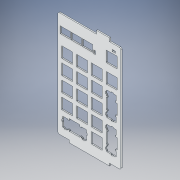
# Autodesk Inventor part: NumpadPlate
Saved by Autodesk Inventor 2018 (Build 220112000, 112)
## iProperties
Created: 2024-10-28
Part Number: NumpadPlate
Material: Generic
Document SubType Name: Modeling
Designer: yuchi
Density: 1 g/cm^3
Appearance: White
Author: yuchi
Autodesk Inventor part; units mm, degrees
ref_plane "YZ Plane" through (0, 0, 0) normal (1, 0, 0) x (0, 1, 0)
ref_plane "XZ Plane" through (0, 0, 0) normal (0, 1, 0) x (-1, 0, 0)
ref_plane "XY Plane" through (0, 0, 0) normal (0, 0, 1) x (1, 0, 0)
sketch "0" plane through (0, 0, 0) normal (0, 0, 1) x (1, 0, 0)
  line L0 (0.6438, 2.2375) -> (13.6438, 2.2375)
  line L1 (0.6438, -11.7625) -> (13.6438, -11.7625)
  line L2 (0.1438, 1.7375) -> (0.1438, -11.2625)
  line L3 (14.1438, 1.7375) -> (14.1438, -11.2625)
  arc A0 (0.6438, 2.2375) -> (0.1438, 1.7375) centre (0.6438, 1.7375) ccw
  arc A1 (14.1438, 1.7375) -> (13.6438, 2.2375) centre (13.6438, 1.7375) ccw
  arc A2 (0.1438, -11.2625) -> (0.6438, -11.7625) centre (0.6438, -11.2625) ccw
  arc A3 (13.6438, -11.7625) -> (14.1438, -11.2625) centre (13.6438, -11.2625) ccw
  line L4 (14.9313, 2.2375) -> (27.9312, 2.2375)
  line L5 (14.9313, -11.7625) -> (27.9312, -11.7625)
  line L6 (14.4313, 1.7375) -> (14.4313, -11.2625)
  line L7 (28.4313, 1.7375) -> (28.4313, -11.2625)
  arc A4 (14.9313, 2.2375) -> (14.4313, 1.7375) centre (14.9313, 1.7375) ccw
  arc A5 (28.4313, 1.7375) -> (27.9312, 2.2375) centre (27.9312, 1.7375) ccw
  arc A6 (14.4313, -11.2625) -> (14.9313, -11.7625) centre (14.9313, -11.2625) ccw
  arc A7 (27.9312, -11.7625) -> (28.4313, -11.2625) centre (27.9312, -11.2625) ccw
  line L8 (29.2188, 2.2375) -> (42.2188, 2.2375)
  line L9 (29.2188, -11.7625) -> (42.2188, -11.7625)
  line L10 (28.7188, 1.7375) -> (28.7188, -11.2625)
  line L11 (42.7188, 1.7375) -> (42.7188, -11.2625)
  arc A8 (29.2188, 2.2375) -> (28.7188, 1.7375) centre (29.2188, 1.7375) ccw
  arc A9 (42.7188, 1.7375) -> (42.2188, 2.2375) centre (42.2188, 1.7375) ccw
  arc A10 (28.7188, -11.2625) -> (29.2188, -11.7625) centre (29.2188, -11.2625) ccw
  arc A11 (42.2188, -11.7625) -> (42.7188, -11.2625) centre (42.2188, -11.2625) ccw
  line L12 (3.025, -21.575) -> (16.025, -21.575)
  line L13 (3.025, -35.575) -> (16.025, -35.575)
  line L14 (2.525, -22.075) -> (2.525, -35.075)
  line L15 (16.525, -22.075) -> (16.525, -35.075)
  arc A12 (3.025, -21.575) -> (2.525, -22.075) centre (3.025, -22.075) ccw
  arc A13 (16.525, -22.075) -> (16.025, -21.575) centre (16.025, -22.075) ccw
  arc A14 (2.525, -35.075) -> (3.025, -35.575) centre (3.025, -35.075) ccw
  arc A15 (16.025, -35.575) -> (16.525, -35.075) centre (16.025, -35.075) ccw
  line L16 (22.075, -21.575) -> (35.075, -21.575)
  line L17 (22.075, -35.575) -> (35.075, -35.575)
  line L18 (21.575, -22.075) -> (21.575, -35.075)
  line L19 (35.575, -22.075) -> (35.575, -35.075)
  arc A16 (22.075, -21.575) -> (21.575, -22.075) centre (22.075, -22.075) ccw
  arc A17 (35.575, -22.075) -> (35.075, -21.575) centre (35.075, -22.075) ccw
  arc A18 (21.575, -35.075) -> (22.075, -35.575) centre (22.075, -35.075) ccw
  arc A19 (35.075, -35.575) -> (35.575, -35.075) centre (35.075, -35.075) ccw
  line L20 (41.125, -21.575) -> (54.125, -21.575)
  line L21 (41.125, -35.575) -> (54.125, -35.575)
  line L22 (40.625, -22.075) -> (40.625, -35.075)
  line L23 (54.625, -22.075) -> (54.625, -35.075)
  arc A20 (41.125, -21.575) -> (40.625, -22.075) centre (41.125, -22.075) ccw
  arc A21 (54.625, -22.075) -> (54.125, -21.575) centre (54.125, -22.075) ccw
  arc A22 (40.625, -35.075) -> (41.125, -35.575) centre (41.125, -35.075) ccw
  arc A23 (54.125, -35.575) -> (54.625, -35.075) centre (54.125, -35.075) ccw
  line L24 (60.175, -21.575) -> (73.175, -21.575)
  line L25 (60.175, -35.575) -> (73.175, -35.575)
  line L26 (59.675, -22.075) -> (59.675, -35.075)
  line L27 (73.675, -22.075) -> (73.675, -35.075)
  arc A24 (60.175, -21.575) -> (59.675, -22.075) centre (60.175, -22.075) ccw
  arc A25 (73.675, -22.075) -> (73.175, -21.575) centre (73.175, -22.075) ccw
  arc A26 (59.675, -35.075) -> (60.175, -35.575) centre (60.175, -35.075) ccw
  arc A27 (73.175, -35.575) -> (73.675, -35.075) centre (73.175, -35.075) ccw
  line L28 (3.025, -40.625) -> (16.025, -40.625)
  line L29 (3.025, -54.625) -> (16.025, -54.625)
  line L30 (2.525, -41.125) -> (2.525, -54.125)
  line L31 (16.525, -41.125) -> (16.525, -54.125)
  arc A28 (3.025, -40.625) -> (2.525, -41.125) centre (3.025, -41.125) ccw
  arc A29 (16.525, -41.125) -> (16.025, -40.625) centre (16.025, -41.125) ccw
  arc A30 (2.525, -54.125) -> (3.025, -54.625) centre (3.025, -54.125) ccw
  arc A31 (16.025, -54.625) -> (16.525, -54.125) centre (16.025, -54.125) ccw
  line L32 (22.075, -40.625) -> (35.075, -40.625)
  line L33 (22.075, -54.625) -> (35.075, -54.625)
  line L34 (21.575, -41.125) -> (21.575, -54.125)
  line L35 (35.575, -41.125) -> (35.575, -54.125)
  arc A32 (22.075, -40.625) -> (21.575, -41.125) centre (22.075, -41.125) ccw
  arc A33 (35.575, -41.125) -> (35.075, -40.625) centre (35.075, -41.125) ccw
  arc A34 (21.575, -54.125) -> (22.075, -54.625) centre (22.075, -54.125) ccw
  arc A35 (35.075, -54.625) -> (35.575, -54.125) centre (35.075, -54.125) ccw
  line L36 (41.125, -40.625) -> (54.125, -40.625)
  line L37 (41.125, -54.625) -> (54.125, -54.625)
  line L38 (40.625, -41.125) -> (40.625, -54.125)
  line L39 (54.625, -41.125) -> (54.625, -54.125)
  arc A36 (41.125, -40.625) -> (40.625, -41.125) centre (41.125, -41.125) ccw
  arc A37 (54.625, -41.125) -> (54.125, -40.625) centre (54.125, -41.125) ccw
  arc A38 (40.625, -54.125) -> (41.125, -54.625) centre (41.125, -54.125) ccw
  arc A39 (54.125, -54.625) -> (54.625, -54.125) centre (54.125, -54.125) ccw
  line L40 (73.675, -50.65) -> (73.675, -63.65)
  line L41 (59.675, -50.65) -> (59.675, -63.65)
  line L42 (73.175, -50.15) -> (60.175, -50.15)
  line L43 (73.175, -64.15) -> (60.175, -64.15)
  arc A40 (73.675, -50.65) -> (73.175, -50.15) centre (73.175, -50.65) ccw
  arc A41 (73.175, -64.15) -> (73.675, -63.65) centre (73.175, -63.65) ccw
  arc A42 (60.175, -50.15) -> (59.675, -50.65) centre (60.175, -50.65) ccw
  arc A43 (59.675, -63.65) -> (60.175, -64.15) centre (60.175, -63.65) ccw
  line L44 (72.3646, -42.3846) -> (72.3646, -48.0394)
  line L45 (71.8646, -48.5394) -> (71.5518, -48.5394)
  line L46 (71.5518, -48.5394) -> (71.5518, -57.15)
  line L47 (60.8584, -57.15) -> (60.8584, -49.0394)
  line L48 (60.3584, -48.5394) -> (60.071, -48.5394)
  line L49 (60.071, -48.5394) -> (60.071, -47.236)
  line L50 (59.571, -46.736) -> (59.4026, -46.736)
  line L51 (58.9026, -46.236) -> (58.9026, -44.188)
  line L52 (59.4026, -43.688) -> (59.571, -43.688)
  line L53 (60.071, -43.188) -> (60.071, -42.3846)
  line L54 (60.571, -41.8846) -> (65.667, -41.8846)
  line L55 (66.167, -41.3846) -> (66.167, -41.021)
  line L56 (66.167, -41.021) -> (68.461, -41.021)
  line L57 (68.961, -41.521) -> (68.961, -41.8846)
  line L58 (68.961, -41.8846) -> (71.8646, -41.8846)
  arc A44 (71.8646, -48.5394) -> (72.3646, -48.0394) centre (71.8646, -48.0394) ccw
  arc A45 (60.8584, -49.0394) -> (60.3584, -48.5394) centre (60.3584, -49.0394) ccw
  arc A46 (60.071, -47.236) -> (59.571, -46.736) centre (59.571, -47.236) ccw
  arc A47 (58.9026, -46.236) -> (59.4026, -46.736) centre (59.4026, -46.236) ccw
  arc A48 (59.4026, -43.688) -> (58.9026, -44.188) centre (59.4026, -44.188) ccw
  arc A49 (59.571, -43.688) -> (60.071, -43.188) centre (59.571, -43.188) ccw
  arc A50 (60.571, -41.8846) -> (60.071, -42.3846) centre (60.571, -42.3846) ccw
  arc A51 (65.667, -41.8846) -> (66.167, -41.3846) centre (65.667, -41.3846) ccw
  arc A52 (68.961, -41.521) -> (68.461, -41.021) centre (68.461, -41.521) ccw
  arc A53 (72.3646, -42.3846) -> (71.8646, -41.8846) centre (71.8646, -42.3846) ccw
  line L59 (72.3646, -71.9154) -> (72.3646, -66.2606)
  line L60 (71.8646, -65.7606) -> (71.5518, -65.7606)
  line L61 (71.5518, -65.7606) -> (71.5518, -57.15)
  line L62 (60.8584, -57.15) -> (60.8584, -65.2606)
  line L63 (60.3584, -65.7606) -> (60.071, -65.7606)
  line L64 (60.071, -65.7606) -> (60.071, -67.064)
  line L65 (59.571, -67.564) -> (59.4026, -67.564)
  line L66 (58.9026, -68.064) -> (58.9026, -70.112)
  line L67 (59.4026, -70.612) -> (59.571, -70.612)
  line L68 (60.071, -71.112) -> (60.071, -71.9154)
  line L69 (60.571, -72.4154) -> (65.667, -72.4154)
  line L70 (66.167, -72.9154) -> (66.167, -73.279)
  line L71 (66.167, -73.279) -> (68.461, -73.279)
  line L72 (68.961, -72.779) -> (68.961, -72.4154)
  line L73 (68.961, -72.4154) -> (71.8646, -72.4154)
  arc A54 (72.3646, -66.2606) -> (71.8646, -65.7606) centre (71.8646, -66.2606) ccw
  arc A55 (60.3584, -65.7606) -> (60.8584, -65.2606) centre (60.3584, -65.2606) ccw
  arc A56 (59.571, -67.564) -> (60.071, -67.064) centre (59.571, -67.064) ccw
  arc A57 (59.4026, -67.564) -> (58.9026, -68.064) centre (59.4026, -68.064) ccw
  arc A58 (58.9026, -70.112) -> (59.4026, -70.612) centre (59.4026, -70.112) ccw
  arc A59 (60.071, -71.112) -> (59.571, -70.612) centre (59.571, -71.112) ccw
  arc A60 (60.071, -71.9154) -> (60.571, -72.4154) centre (60.571, -71.9154) ccw
  arc A61 (66.167, -72.9154) -> (65.667, -72.4154) centre (65.667, -72.9154) ccw
  arc A62 (68.461, -73.279) -> (68.961, -72.779) centre (68.461, -72.779) ccw
  arc A63 (71.8646, -72.4154) -> (72.3646, -71.9154) centre (71.8646, -71.9154) ccw
  line L74 (3.025, -59.675) -> (16.025, -59.675)
  line L75 (3.025, -73.675) -> (16.025, -73.675)
  line L76 (2.525, -60.175) -> (2.525, -73.175)
  line L77 (16.525, -60.175) -> (16.525, -73.175)
  arc A64 (3.025, -59.675) -> (2.525, -60.175) centre (3.025, -60.175) ccw
  arc A65 (16.525, -60.175) -> (16.025, -59.675) centre (16.025, -60.175) ccw
  arc A66 (2.525, -73.175) -> (3.025, -73.675) centre (3.025, -73.175) ccw
  arc A67 (16.025, -73.675) -> (16.525, -73.175) centre (16.025, -73.175) ccw
  line L78 (22.075, -59.675) -> (35.075, -59.675)
  line L79 (22.075, -73.675) -> (35.075, -73.675)
  line L80 (21.575, -60.175) -> (21.575, -73.175)
  line L81 (35.575, -60.175) -> (35.575, -73.175)
  arc A68 (22.075, -59.675) -> (21.575, -60.175) centre (22.075, -60.175) ccw
  arc A69 (35.575, -60.175) -> (35.075, -59.675) centre (35.075, -60.175) ccw
  arc A70 (21.575, -73.175) -> (22.075, -73.675) centre (22.075, -73.175) ccw
  arc A71 (35.075, -73.675) -> (35.575, -73.175) centre (35.075, -73.175) ccw
  line L82 (41.125, -59.675) -> (54.125, -59.675)
  line L83 (41.125, -73.675) -> (54.125, -73.675)
  line L84 (40.625, -60.175) -> (40.625, -73.175)
  line L85 (54.625, -60.175) -> (54.625, -73.175)
  arc A72 (41.125, -59.675) -> (40.625, -60.175) centre (41.125, -60.175) ccw
  arc A73 (54.625, -60.175) -> (54.125, -59.675) centre (54.125, -60.175) ccw
  arc A74 (40.625, -73.175) -> (41.125, -73.675) centre (41.125, -73.175) ccw
  arc A75 (54.125, -73.675) -> (54.625, -73.175) centre (54.125, -73.175) ccw
  line L86 (3.025, -78.725) -> (16.025, -78.725)
  line L87 (3.025, -92.725) -> (16.025, -92.725)
  line L88 (2.525, -79.225) -> (2.525, -92.225)
  line L89 (16.525, -79.225) -> (16.525, -92.225)
  arc A76 (3.025, -78.725) -> (2.525, -79.225) centre (3.025, -79.225) ccw
  arc A77 (16.525, -79.225) -> (16.025, -78.725) centre (16.025, -79.225) ccw
  arc A78 (2.525, -92.225) -> (3.025, -92.725) centre (3.025, -92.225) ccw
  arc A79 (16.025, -92.725) -> (16.525, -92.225) centre (16.025, -92.225) ccw
  line L90 (22.075, -78.725) -> (35.075, -78.725)
  line L91 (22.075, -92.725) -> (35.075, -92.725)
  line L92 (21.575, -79.225) -> (21.575, -92.225)
  line L93 (35.575, -79.225) -> (35.575, -92.225)
  arc A80 (22.075, -78.725) -> (21.575, -79.225) centre (22.075, -79.225) ccw
  arc A81 (35.575, -79.225) -> (35.075, -78.725) centre (35.075, -79.225) ccw
  arc A82 (21.575, -92.225) -> (22.075, -92.725) centre (22.075, -92.225) ccw
  arc A83 (35.075, -92.725) -> (35.575, -92.225) centre (35.075, -92.225) ccw
  line L94 (41.125, -78.725) -> (54.125, -78.725)
  line L95 (41.125, -92.725) -> (54.125, -92.725)
  line L96 (40.625, -79.225) -> (40.625, -92.225)
  line L97 (54.625, -79.225) -> (54.625, -92.225)
  arc A84 (41.125, -78.725) -> (40.625, -79.225) centre (41.125, -79.225) ccw
  arc A85 (54.625, -79.225) -> (54.125, -78.725) centre (54.125, -79.225) ccw
  arc A86 (40.625, -92.225) -> (41.125, -92.725) centre (41.125, -92.225) ccw
  arc A87 (54.125, -92.725) -> (54.625, -92.225) centre (54.125, -92.225) ccw
  line L98 (73.675, -88.75) -> (73.675, -101.75)
  line L99 (59.675, -88.75) -> (59.675, -101.75)
  line L100 (73.175, -88.25) -> (60.175, -88.25)
  line L101 (73.175, -102.25) -> (60.175, -102.25)
  arc A88 (73.675, -88.75) -> (73.175, -88.25) centre (73.175, -88.75) ccw
  arc A89 (73.175, -102.25) -> (73.675, -101.75) centre (73.175, -101.75) ccw
  arc A90 (60.175, -88.25) -> (59.675, -88.75) centre (60.175, -88.75) ccw
  arc A91 (59.675, -101.75) -> (60.175, -102.25) centre (60.175, -101.75) ccw
  line L102 (72.3646, -80.4846) -> (72.3646, -86.1394)
  line L103 (71.8646, -86.6394) -> (71.5518, -86.6394)
  line L104 (71.5518, -86.6394) -> (71.5518, -95.25)
  line L105 (60.8584, -95.25) -> (60.8584, -87.1394)
  line L106 (60.3584, -86.6394) -> (60.071, -86.6394)
  line L107 (60.071, -86.6394) -> (60.071, -85.336)
  line L108 (59.571, -84.836) -> (59.4026, -84.836)
  line L109 (58.9026, -84.336) -> (58.9026, -82.288)
  line L110 (59.4026, -81.788) -> (59.571, -81.788)
  line L111 (60.071, -81.288) -> (60.071, -80.4846)
  line L112 (60.571, -79.9846) -> (65.667, -79.9846)
  line L113 (66.167, -79.4846) -> (66.167, -79.121)
  line L114 (66.167, -79.121) -> (68.461, -79.121)
  line L115 (68.961, -79.621) -> (68.961, -79.9846)
  line L116 (68.961, -79.9846) -> (71.8646, -79.9846)
  arc A92 (71.8646, -86.6394) -> (72.3646, -86.1394) centre (71.8646, -86.1394) ccw
  arc A93 (60.8584, -87.1394) -> (60.3584, -86.6394) centre (60.3584, -87.1394) ccw
  arc A94 (60.071, -85.336) -> (59.571, -84.836) centre (59.571, -85.336) ccw
  arc A95 (58.9026, -84.336) -> (59.4026, -84.836) centre (59.4026, -84.336) ccw
  arc A96 (59.4026, -81.788) -> (58.9026, -82.288) centre (59.4026, -82.288) ccw
  arc A97 (59.571, -81.788) -> (60.071, -81.288) centre (59.571, -81.288) ccw
  arc A98 (60.571, -79.9846) -> (60.071, -80.4846) centre (60.571, -80.4846) ccw
  arc A99 (65.667, -79.9846) -> (66.167, -79.4846) centre (65.667, -79.4846) ccw
  arc A100 (68.961, -79.621) -> (68.461, -79.121) centre (68.461, -79.621) ccw
  arc A101 (72.3646, -80.4846) -> (71.8646, -79.9846) centre (71.8646, -80.4846) ccw
  line L117 (72.3646, -110.0154) -> (72.3646, -104.3606)
  line L118 (71.8646, -103.8606) -> (71.5518, -103.8606)
  line L119 (71.5518, -103.8606) -> (71.5518, -95.25)
  line L120 (60.8584, -95.25) -> (60.8584, -103.3606)
  line L121 (60.3584, -103.8606) -> (60.071, -103.8606)
  line L122 (60.071, -103.8606) -> (60.071, -105.164)
  line L123 (59.571, -105.664) -> (59.4026, -105.664)
  line L124 (58.9026, -106.164) -> (58.9026, -108.212)
  line L125 (59.4026, -108.712) -> (59.571, -108.712)
  line L126 (60.071, -109.212) -> (60.071, -110.0154)
  line L127 (60.571, -110.5154) -> (65.667, -110.5154)
  line L128 (66.167, -111.0154) -> (66.167, -111.379)
  line L129 (66.167, -111.379) -> (68.461, -111.379)
  line L130 (68.961, -110.879) -> (68.961, -110.5154)
  line L131 (68.961, -110.5154) -> (71.8646, -110.5154)
  arc A102 (72.3646, -104.3606) -> (71.8646, -103.8606) centre (71.8646, -104.3606) ccw
  arc A103 (60.3584, -103.8606) -> (60.8584, -103.3606) centre (60.3584, -103.3606) ccw
  arc A104 (59.571, -105.664) -> (60.071, -105.164) centre (59.571, -105.164) ccw
  arc A105 (59.4026, -105.664) -> (58.9026, -106.164) centre (59.4026, -106.164) ccw
  arc A106 (58.9026, -108.212) -> (59.4026, -108.712) centre (59.4026, -108.212) ccw
  arc A107 (60.071, -109.212) -> (59.571, -108.712) centre (59.571, -109.212) ccw
  arc A108 (60.071, -110.0154) -> (60.571, -110.5154) centre (60.571, -110.0154) ccw
  arc A109 (66.167, -111.0154) -> (65.667, -110.5154) centre (65.667, -111.0154) ccw
  arc A110 (68.461, -111.379) -> (68.961, -110.879) centre (68.461, -110.879) ccw
  arc A111 (71.8646, -110.5154) -> (72.3646, -110.0154) centre (71.8646, -110.0154) ccw
  line L132 (12.55, -97.775) -> (25.55, -97.775)
  line L133 (12.55, -111.775) -> (25.55, -111.775)
  line L134 (12.05, -98.275) -> (12.05, -111.275)
  line L135 (26.05, -98.275) -> (26.05, -111.275)
  arc A112 (12.55, -97.775) -> (12.05, -98.275) centre (12.55, -98.275) ccw
  arc A113 (26.05, -98.275) -> (25.55, -97.775) centre (25.55, -98.275) ccw
  arc A114 (12.05, -111.275) -> (12.55, -111.775) centre (12.55, -111.275) ccw
  arc A115 (25.55, -111.775) -> (26.05, -111.275) centre (25.55, -111.275) ccw
  line L136 (4.2846, -99.0854) -> (9.9394, -99.0854)
  line L137 (10.4394, -99.5854) -> (10.4394, -99.8982)
  line L138 (10.4394, -99.8982) -> (19.05, -99.8982)
  line L139 (19.05, -110.5916) -> (10.9394, -110.5916)
  line L140 (10.4394, -111.0916) -> (10.4394, -111.379)
  line L141 (10.4394, -111.379) -> (9.136, -111.379)
  line L142 (8.636, -111.879) -> (8.636, -112.0474)
  line L143 (8.136, -112.5474) -> (6.088, -112.5474)
  line L144 (5.588, -112.0474) -> (5.588, -111.879)
  line L145 (5.088, -111.379) -> (4.2846, -111.379)
  line L146 (3.7846, -110.879) -> (3.7846, -105.783)
  line L147 (3.2846, -105.283) -> (2.921, -105.283)
  line L148 (2.921, -105.283) -> (2.921, -102.989)
  line L149 (3.421, -102.489) -> (3.7846, -102.489)
  line L150 (3.7846, -102.489) -> (3.7846, -99.5854)
  arc A116 (10.4394, -99.5854) -> (9.9394, -99.0854) centre (9.9394, -99.5854) ccw
  arc A117 (10.9394, -110.5916) -> (10.4394, -111.0916) centre (10.9394, -111.0916) ccw
  arc A118 (9.136, -111.379) -> (8.636, -111.879) centre (9.136, -111.879) ccw
  arc A119 (8.136, -112.5474) -> (8.636, -112.0474) centre (8.136, -112.0474) ccw
  arc A120 (5.588, -112.0474) -> (6.088, -112.5474) centre (6.088, -112.0474) ccw
  arc A121 (5.588, -111.879) -> (5.088, -111.379) centre (5.088, -111.879) ccw
  arc A122 (3.7846, -110.879) -> (4.2846, -111.379) centre (4.2846, -110.879) ccw
  arc A123 (3.7846, -105.783) -> (3.2846, -105.283) centre (3.2846, -105.783) ccw
  arc A124 (3.421, -102.489) -> (2.921, -102.989) centre (3.421, -102.989) ccw
  arc A125 (4.2846, -99.0854) -> (3.7846, -99.5854) centre (4.2846, -99.5854) ccw
  line L151 (33.8154, -99.0854) -> (28.1606, -99.0854)
  line L152 (27.6606, -99.5854) -> (27.6606, -99.8982)
  line L153 (27.6606, -99.8982) -> (19.05, -99.8982)
  line L154 (19.05, -110.5916) -> (27.1606, -110.5916)
  line L155 (27.6606, -111.0916) -> (27.6606, -111.379)
  line L156 (27.6606, -111.379) -> (28.964, -111.379)
  line L157 (29.464, -111.879) -> (29.464, -112.0474)
  line L158 (29.964, -112.5474) -> (32.012, -112.5474)
  line L159 (32.512, -112.0474) -> (32.512, -111.879)
  line L160 (33.012, -111.379) -> (33.8154, -111.379)
  line L161 (34.3154, -110.879) -> (34.3154, -105.783)
  line L162 (34.8154, -105.283) -> (35.179, -105.283)
  line L163 (35.179, -105.283) -> (35.179, -102.989)
  line L164 (34.679, -102.489) -> (34.3154, -102.489)
  line L165 (34.3154, -102.489) -> (34.3154, -99.5854)
  arc A126 (28.1606, -99.0854) -> (27.6606, -99.5854) centre (28.1606, -99.5854) ccw
  arc A127 (27.6606, -111.0916) -> (27.1606, -110.5916) centre (27.1606, -111.0916) ccw
  arc A128 (29.464, -111.879) -> (28.964, -111.379) centre (28.964, -111.879) ccw
  arc A129 (29.464, -112.0474) -> (29.964, -112.5474) centre (29.964, -112.0474) ccw
  arc A130 (32.012, -112.5474) -> (32.512, -112.0474) centre (32.012, -112.0474) ccw
  arc A131 (33.012, -111.379) -> (32.512, -111.879) centre (33.012, -111.879) ccw
  arc A132 (33.8154, -111.379) -> (34.3154, -110.879) centre (33.8154, -110.879) ccw
  arc A133 (34.8154, -105.283) -> (34.3154, -105.783) centre (34.8154, -105.783) ccw
  arc A134 (35.179, -102.989) -> (34.679, -102.489) centre (34.679, -102.989) ccw
  arc A135 (34.3154, -99.5854) -> (33.8154, -99.0854) centre (33.8154, -99.5854) ccw
  line L166 (41.125, -97.775) -> (54.125, -97.775)
  line L167 (41.125, -111.775) -> (54.125, -111.775)
  line L168 (40.625, -98.275) -> (40.625, -111.275)
  line L169 (54.625, -98.275) -> (54.625, -111.275)
  arc A136 (41.125, -97.775) -> (40.625, -98.275) centre (41.125, -98.275) ccw
  arc A137 (54.625, -98.275) -> (54.125, -97.775) centre (54.125, -98.275) ccw
  arc A138 (40.625, -111.275) -> (41.125, -111.775) centre (41.125, -111.275) ccw
  arc A139 (54.125, -111.775) -> (54.625, -111.275) centre (54.125, -111.275) ccw
  line L170 (0, -114.3) -> (76.2, -114.3)
  line L171 (0, 0) -> (76.2, 0)
  line L172 (0, -114.3) -> (0, 0)
  line L173 (76.2, -114.3) -> (76.2, 0)
  dimension "d31" = 14
  dimension "d32" = 14
  constraints: 348 end point, 280 point on circle, 140 centre point
  measures "d31" distance between parallel lines of L25 L24
  measures "d32" distance between parallel lines of L27 L26
extrude "Extrusion1" add sketch "0" along normal blind 1.6 contours L171 L3 A3 L1 A2 L2 | L2 A2 L1 A3 L3 L171 L6 A6 L5 A7 L7 L10 A10 L9 A11 L11 L173 L170 L172 | L171 L7 A7 L5 A6 L6 | L171 L11 A11 L9 A10 L10
sketch "Sketch3" plane through (0, 0, 1.6) normal (0, 0, 1) x (1, 0, 0)
  line L0 (76.2, 0) -> (0, 0) projected
  line L1 (3.025, -21.575) -> (16.025, -21.575) projected
  line L2 (0.545, -9.117) -> (13.746, -9.117)
  line L3 (13.746, -9.117) -> (13.746, -0.408)
  line L4 (13.746, -0.408) -> (0.545, -0.408)
  line L5 (0.545, -0.408) -> (0.545, -9.117)
  line L6 (16.025, -21.575) -> (3.025, -21.575) projected
  line L7 (16.525, -22.075) -> (16.525, -35.075) projected
  line L8 (14.829, -0.408) -> (28.03, -0.408)
  line L9 (28.03, -0.408) -> (28.03, -9.117)
  line L10 (28.03, -9.117) -> (14.829, -9.117)
  line L11 (14.829, -9.117) -> (14.829, -0.408)
  line L12 (29.113, -0.408) -> (42.314, -0.408)
  line L13 (42.314, -0.408) -> (42.314, -9.117)
  line L14 (42.314, -9.117) -> (29.113, -9.117)
  line L15 (29.113, -9.117) -> (29.113, -0.408)
  point P0 (9.525, -21.575)
  point P1 (16.525, -28.575)
  dimension "d9" = 13.201
  dimension "d10" = 8.709
  dimension "d11" = 4.221
  dimension "d12" = 19.458
  dimension "d19" = 13.201
  dimension "d20" = 1.083
  dimension "d21" = 13.201
  dimension "d22" = 1.083
  constraints: 24 end point, 6 parallel, 3 horizontal, 3 perpendicular, 2 midpoint
  measures "d9" distance of L2.start L2.end
  measures "d10" distance of L2.end L3.end
  measures "d11" horizontal distance of point (9.525, -21.575) L2.end
  measures "d12" vertical distance of L2.end point (16.525, -28.575)
  measures "d19" distance between parallel lines of L9 L11
  measures "d20" distance between parallel lines of L11 L3
  measures "d21" distance of L13.end L14.end
  measures "d22" distance between parallel lines of L9 L15
extrude "Extrusion2" cut sketch "Sketch3" against normal blind 1.6
sketch "Sketch6" plane through (0, -114.3, 0) normal (-1, 0, 0) x (0, 0, 1)
  line L0 (0, 0) -> (0, 114.3) projected
  line L1 (0, 0) -> (1.6, 0) projected
  line L2 (1.6, 114.3) -> (1.6, 0) projected
  line L3 (0, 114.3) -> (1.6, 114.3) projected
extrude "Extrusion3" add sketch "Sketch6" along normal blind 2.381
sketch "Sketch7" plane through (76.2, -114.3, 0) normal (1, 0, 0) x (0, 0, -1)
  line L0 (0, 114.3) -> (0, 0) projected
  line L1 (0, 114.3) -> (-1.6, 114.3) projected
  line L2 (-1.6, 0) -> (-1.6, 114.3) projected
  line L3 (0, 0) -> (-1.6, 0) projected
extrude "Extrusion4" add sketch "Sketch7" along normal blind 2.381
sketch "Sketch9" plane through (-2.381, 0, 0) normal (0, 1, 0) x (1, 0, 0)
  line L0 (0, 0) -> (80.962, 0) projected
  line L1 (0, -1.6) -> (0, 0) projected
  line L2 (0, -1.6) -> (80.962, -1.6) projected
  line L3 (80.962, 0) -> (80.962, -1.6) projected
  point P0 (2.381, 0)
extrude "Extrusion5" add sketch "Sketch9" along normal blind 13.517
sketch "Sketch11" plane through (-2.381, -114.3, 0) normal (0, -1, 0) x (1, 0, 0)
  line L0 (80.962, 0) -> (0, 0) projected
  line L1 (80.962, 1.6) -> (80.962, 0) projected
  line L2 (80.962, 1.6) -> (0, 1.6) projected
  line L3 (0, 0) -> (0, 1.6) projected
  point P0 (2.381, 0)
extrude "Extrusion6" add sketch "Sketch11" along normal blind 7.183
sketch "Sketch12" plane through (0, 0, 1.6) normal (0, 0, 1) x (1, 0, 0)
  line L0 (14.829, -9.117) -> (14.829, -0.408) projected
  line L1 (14.829, -0.408) -> (28.03, -0.408) projected
  line L2 (28.03, -0.408) -> (28.03, -9.117) projected
  line L3 (28.03, -9.117) -> (14.829, -9.117) projected
  line L4 (13.746, -0.408) -> (13.746, -9.117) projected
  line L5 (13.746, -9.117) -> (0.545, -9.117) projected
  line L6 (0.545, -9.117) -> (0.545, -0.408) projected
  line L7 (0.545, -0.408) -> (13.746, -0.408) projected
  line L8 (29.113, -9.117) -> (29.113, -0.408) projected
  line L9 (29.113, -0.408) -> (42.314, -0.408) projected
  line L10 (42.314, -0.408) -> (42.314, -9.117) projected
  line L11 (42.314, -9.117) -> (29.113, -9.117) projected
  line L12 (71.5518, -102.25) -> (71.5518, -103.8606) projected
  line L13 (71.5518, -103.8606) -> (71.8646, -103.8606) projected
  arc A0 (72.3646, -104.3606) -> (71.8646, -103.8606) centre (71.8646, -104.3606) ccw projected
  line L14 (72.3646, -104.3606) -> (72.3646, -110.0154) projected
  arc A1 (71.8646, -110.5154) -> (72.3646, -110.0154) centre (71.8646, -110.0154) ccw projected
  line L15 (71.8646, -110.5154) -> (68.961, -110.5154) projected
  line L16 (68.961, -110.5154) -> (68.961, -110.879) projected
  arc A2 (68.461, -111.379) -> (68.961, -110.879) centre (68.461, -110.879) ccw projected
  line L17 (68.461, -111.379) -> (66.167, -111.379) projected
  line L18 (66.167, -111.379) -> (66.167, -111.0154) projected
  arc A3 (66.167, -111.0154) -> (65.667, -110.5154) centre (65.667, -111.0154) ccw projected
  line L19 (65.667, -110.5154) -> (60.571, -110.5154) projected
  arc A4 (60.071, -110.0154) -> (60.571, -110.5154) centre (60.571, -110.0154) ccw projected
  line L20 (60.071, -110.0154) -> (60.071, -109.212) projected
  arc A5 (60.071, -109.212) -> (59.571, -108.712) centre (59.571, -109.212) ccw projected
  line L21 (59.571, -108.712) -> (59.4026, -108.712) projected
  arc A6 (58.9026, -108.212) -> (59.4026, -108.712) centre (59.4026, -108.212) ccw projected
  line L22 (58.9026, -108.212) -> (58.9026, -106.164) projected
  arc A7 (59.4026, -105.664) -> (58.9026, -106.164) centre (59.4026, -106.164) ccw projected
  line L23 (59.4026, -105.664) -> (59.571, -105.664) projected
  arc A8 (59.571, -105.664) -> (60.071, -105.164) centre (59.571, -105.164) ccw projected
  line L24 (60.071, -105.164) -> (60.071, -103.8606) projected
  line L25 (60.071, -103.8606) -> (60.3584, -103.8606) projected
  arc A9 (60.3584, -103.8606) -> (60.8584, -103.3606) centre (60.3584, -103.3606) ccw projected
  line L26 (60.8584, -103.3606) -> (60.8584, -102.25) projected
  line L27 (60.8584, -102.25) -> (60.175, -102.25) projected
  arc A10 (59.675, -101.75) -> (60.175, -102.25) centre (60.175, -101.75) ccw projected
  line L28 (59.675, -101.75) -> (59.675, -88.75) projected
  arc A11 (60.175, -88.25) -> (59.675, -88.75) centre (60.175, -88.75) ccw projected
  line L29 (60.175, -88.25) -> (60.8584, -88.25) projected
  line L30 (60.8584, -88.25) -> (60.8584, -87.1394) projected
  arc A12 (60.8584, -87.1394) -> (60.3584, -86.6394) centre (60.3584, -87.1394) ccw projected
  line L31 (60.3584, -86.6394) -> (60.071, -86.6394) projected
  line L32 (60.071, -86.6394) -> (60.071, -85.336) projected
  arc A13 (60.071, -85.336) -> (59.571, -84.836) centre (59.571, -85.336) ccw projected
  line L33 (59.571, -84.836) -> (59.4026, -84.836) projected
  arc A14 (58.9026, -84.336) -> (59.4026, -84.836) centre (59.4026, -84.336) ccw projected
  line L34 (58.9026, -84.336) -> (58.9026, -82.288) projected
  arc A15 (59.4026, -81.788) -> (58.9026, -82.288) centre (59.4026, -82.288) ccw projected
  line L35 (59.4026, -81.788) -> (59.571, -81.788) projected
  arc A16 (59.571, -81.788) -> (60.071, -81.288) centre (59.571, -81.288) ccw projected
  line L36 (60.071, -81.288) -> (60.071, -80.4846) projected
  arc A17 (60.571, -79.9846) -> (60.071, -80.4846) centre (60.571, -80.4846) ccw projected
  line L37 (60.571, -79.9846) -> (65.667, -79.9846) projected
  arc A18 (65.667, -79.9846) -> (66.167, -79.4846) centre (65.667, -79.4846) ccw projected
  line L38 (66.167, -79.4846) -> (66.167, -79.121) projected
  line L39 (66.167, -79.121) -> (68.461, -79.121) projected
  arc A19 (68.961, -79.621) -> (68.461, -79.121) centre (68.461, -79.621) ccw projected
  line L40 (68.961, -79.621) -> (68.961, -79.9846) projected
  line L41 (68.961, -79.9846) -> (71.8646, -79.9846) projected
  arc A20 (72.3646, -80.4846) -> (71.8646, -79.9846) centre (71.8646, -80.4846) ccw projected
  line L42 (72.3646, -80.4846) -> (72.3646, -86.1394) projected
  arc A21 (71.8646, -86.6394) -> (72.3646, -86.1394) centre (71.8646, -86.1394) ccw projected
  line L43 (71.8646, -86.6394) -> (71.5518, -86.6394) projected
  line L44 (71.5518, -86.6394) -> (71.5518, -88.25) projected
  line L45 (71.5518, -88.25) -> (73.175, -88.25) projected
  arc A22 (73.675, -88.75) -> (73.175, -88.25) centre (73.175, -88.75) ccw projected
  line L46 (73.675, -88.75) -> (73.675, -101.75) projected
  arc A23 (73.175, -102.25) -> (73.675, -101.75) centre (73.175, -101.75) ccw projected
  line L47 (73.175, -102.25) -> (71.5518, -102.25) projected
  line L48 (60.8584, -65.2606) -> (60.8584, -64.15) projected
  line L49 (60.8584, -64.15) -> (60.175, -64.15) projected
  arc A24 (59.675, -63.65) -> (60.175, -64.15) centre (60.175, -63.65) ccw projected
  line L50 (59.675, -63.65) -> (59.675, -50.65) projected
  arc A25 (60.175, -50.15) -> (59.675, -50.65) centre (60.175, -50.65) ccw projected
  line L51 (60.175, -50.15) -> (60.8584, -50.15) projected
  line L52 (60.8584, -50.15) -> (60.8584, -49.0394) projected
  arc A26 (60.8584, -49.0394) -> (60.3584, -48.5394) centre (60.3584, -49.0394) ccw projected
  line L53 (60.3584, -48.5394) -> (60.071, -48.5394) projected
  line L54 (60.071, -48.5394) -> (60.071, -47.236) projected
  arc A27 (60.071, -47.236) -> (59.571, -46.736) centre (59.571, -47.236) ccw projected
  line L55 (59.571, -46.736) -> (59.4026, -46.736) projected
  arc A28 (58.9026, -46.236) -> (59.4026, -46.736) centre (59.4026, -46.236) ccw projected
  line L56 (58.9026, -46.236) -> (58.9026, -44.188) projected
  arc A29 (59.4026, -43.688) -> (58.9026, -44.188) centre (59.4026, -44.188) ccw projected
  line L57 (59.4026, -43.688) -> (59.571, -43.688) projected
  arc A30 (59.571, -43.688) -> (60.071, -43.188) centre (59.571, -43.188) ccw projected
  line L58 (60.071, -43.188) -> (60.071, -42.3846) projected
  arc A31 (60.571, -41.8846) -> (60.071, -42.3846) centre (60.571, -42.3846) ccw projected
  line L59 (60.571, -41.8846) -> (65.667, -41.8846) projected
  arc A32 (65.667, -41.8846) -> (66.167, -41.3846) centre (65.667, -41.3846) ccw projected
  line L60 (66.167, -41.3846) -> (66.167, -41.021) projected
  line L61 (66.167, -41.021) -> (68.461, -41.021) projected
  arc A33 (68.961, -41.521) -> (68.461, -41.021) centre (68.461, -41.521) ccw projected
  line L62 (68.961, -41.521) -> (68.961, -41.8846) projected
  line L63 (68.961, -41.8846) -> (71.8646, -41.8846) projected
  arc A34 (72.3646, -42.3846) -> (71.8646, -41.8846) centre (71.8646, -42.3846) ccw projected
  line L64 (72.3646, -42.3846) -> (72.3646, -48.0394) projected
  arc A35 (71.8646, -48.5394) -> (72.3646, -48.0394) centre (71.8646, -48.0394) ccw projected
  line L65 (71.8646, -48.5394) -> (71.5518, -48.5394) projected
  line L66 (71.5518, -48.5394) -> (71.5518, -50.15) projected
  line L67 (71.5518, -50.15) -> (73.175, -50.15) projected
  arc A36 (73.675, -50.65) -> (73.175, -50.15) centre (73.175, -50.65) ccw projected
  line L68 (73.675, -50.65) -> (73.675, -63.65) projected
  arc A37 (73.175, -64.15) -> (73.675, -63.65) centre (73.175, -63.65) ccw projected
  line L69 (73.175, -64.15) -> (71.5518, -64.15) projected
  line L70 (71.5518, -64.15) -> (71.5518, -65.7606) projected
  line L71 (71.5518, -65.7606) -> (71.8646, -65.7606) projected
  arc A38 (72.3646, -66.2606) -> (71.8646, -65.7606) centre (71.8646, -66.2606) ccw projected
  line L72 (72.3646, -66.2606) -> (72.3646, -71.9154) projected
  arc A39 (71.8646, -72.4154) -> (72.3646, -71.9154) centre (71.8646, -71.9154) ccw projected
  line L73 (71.8646, -72.4154) -> (68.961, -72.4154) projected
  line L74 (68.961, -72.4154) -> (68.961, -72.779) projected
  arc A40 (68.461, -73.279) -> (68.961, -72.779) centre (68.461, -72.779) ccw projected
  line L75 (68.461, -73.279) -> (66.167, -73.279) projected
  line L76 (66.167, -73.279) -> (66.167, -72.9154) projected
  arc A41 (66.167, -72.9154) -> (65.667, -72.4154) centre (65.667, -72.9154) ccw projected
  line L77 (65.667, -72.4154) -> (60.571, -72.4154) projected
  arc A42 (60.071, -71.9154) -> (60.571, -72.4154) centre (60.571, -71.9154) ccw projected
  line L78 (60.071, -71.9154) -> (60.071, -71.112) projected
  arc A43 (60.071, -71.112) -> (59.571, -70.612) centre (59.571, -71.112) ccw projected
  line L79 (59.571, -70.612) -> (59.4026, -70.612) projected
  arc A44 (58.9026, -70.112) -> (59.4026, -70.612) centre (59.4026, -70.112) ccw projected
  line L80 (58.9026, -70.112) -> (58.9026, -68.064) projected
  arc A45 (59.4026, -67.564) -> (58.9026, -68.064) centre (59.4026, -68.064) ccw projected
  line L81 (59.4026, -67.564) -> (59.571, -67.564) projected
  arc A46 (59.571, -67.564) -> (60.071, -67.064) centre (59.571, -67.064) ccw projected
  line L82 (60.071, -67.064) -> (60.071, -65.7606) projected
  line L83 (60.071, -65.7606) -> (60.3584, -65.7606) projected
  arc A47 (60.3584, -65.7606) -> (60.8584, -65.2606) centre (60.3584, -65.2606) ccw projected
  line L84 (41.125, -97.775) -> (54.125, -97.775) projected
  arc A48 (54.625, -98.275) -> (54.125, -97.775) centre (54.125, -98.275) ccw projected
  line L85 (54.625, -98.275) -> (54.625, -111.275) projected
  arc A49 (54.125, -111.775) -> (54.625, -111.275) centre (54.125, -111.275) ccw projected
  line L86 (54.125, -111.775) -> (41.125, -111.775) projected
  arc A50 (40.625, -111.275) -> (41.125, -111.775) centre (41.125, -111.275) ccw projected
  line L87 (40.625, -111.275) -> (40.625, -98.275) projected
  arc A51 (41.125, -97.775) -> (40.625, -98.275) centre (41.125, -98.275) ccw projected
  line L88 (41.125, -78.725) -> (54.125, -78.725) projected
  arc A52 (54.625, -79.225) -> (54.125, -78.725) centre (54.125, -79.225) ccw projected
  line L89 (54.625, -79.225) -> (54.625, -92.225) projected
  arc A53 (54.125, -92.725) -> (54.625, -92.225) centre (54.125, -92.225) ccw projected
  line L90 (54.125, -92.725) -> (41.125, -92.725) projected
  arc A54 (40.625, -92.225) -> (41.125, -92.725) centre (41.125, -92.225) ccw projected
  line L91 (40.625, -92.225) -> (40.625, -79.225) projected
  arc A55 (41.125, -78.725) -> (40.625, -79.225) centre (41.125, -79.225) ccw projected
  line L92 (22.075, -78.725) -> (35.075, -78.725) projected
  arc A56 (35.575, -79.225) -> (35.075, -78.725) centre (35.075, -79.225) ccw projected
  line L93 (35.575, -79.225) -> (35.575, -92.225) projected
  arc A57 (35.075, -92.725) -> (35.575, -92.225) centre (35.075, -92.225) ccw projected
  line L94 (35.075, -92.725) -> (22.075, -92.725) projected
  arc A58 (21.575, -92.225) -> (22.075, -92.725) centre (22.075, -92.225) ccw projected
  line L95 (21.575, -92.225) -> (21.575, -79.225) projected
  arc A59 (22.075, -78.725) -> (21.575, -79.225) centre (22.075, -79.225) ccw projected
  line L96 (3.025, -78.725) -> (16.025, -78.725) projected
  arc A60 (16.525, -79.225) -> (16.025, -78.725) centre (16.025, -79.225) ccw projected
  line L97 (16.525, -79.225) -> (16.525, -92.225) projected
  arc A61 (16.025, -92.725) -> (16.525, -92.225) centre (16.025, -92.225) ccw projected
  line L98 (16.025, -92.725) -> (3.025, -92.725) projected
  arc A62 (2.525, -92.225) -> (3.025, -92.725) centre (3.025, -92.225) ccw projected
  line L99 (2.525, -92.225) -> (2.525, -79.225) projected
  arc A63 (3.025, -78.725) -> (2.525, -79.225) centre (3.025, -79.225) ccw projected
  line L100 (41.125, -59.675) -> (54.125, -59.675) projected
  arc A64 (54.625, -60.175) -> (54.125, -59.675) centre (54.125, -60.175) ccw projected
  line L101 (54.625, -60.175) -> (54.625, -73.175) projected
  arc A65 (54.125, -73.675) -> (54.625, -73.175) centre (54.125, -73.175) ccw projected
  line L102 (54.125, -73.675) -> (41.125, -73.675) projected
  arc A66 (40.625, -73.175) -> (41.125, -73.675) centre (41.125, -73.175) ccw projected
  line L103 (40.625, -73.175) -> (40.625, -60.175) projected
  arc A67 (41.125, -59.675) -> (40.625, -60.175) centre (41.125, -60.175) ccw projected
  line L104 (22.075, -59.675) -> (35.075, -59.675) projected
  arc A68 (35.575, -60.175) -> (35.075, -59.675) centre (35.075, -60.175) ccw projected
  line L105 (35.575, -60.175) -> (35.575, -73.175) projected
  arc A69 (35.075, -73.675) -> (35.575, -73.175) centre (35.075, -73.175) ccw projected
  line L106 (35.075, -73.675) -> (22.075, -73.675) projected
  arc A70 (21.575, -73.175) -> (22.075, -73.675) centre (22.075, -73.175) ccw projected
  line L107 (21.575, -73.175) -> (21.575, -60.175) projected
  arc A71 (22.075, -59.675) -> (21.575, -60.175) centre (22.075, -60.175) ccw projected
  line L108 (3.025, -59.675) -> (16.025, -59.675) projected
  arc A72 (16.525, -60.175) -> (16.025, -59.675) centre (16.025, -60.175) ccw projected
  line L109 (16.525, -60.175) -> (16.525, -73.175) projected
  arc A73 (16.025, -73.675) -> (16.525, -73.175) centre (16.025, -73.175) ccw projected
  line L110 (16.025, -73.675) -> (3.025, -73.675) projected
  arc A74 (2.525, -73.175) -> (3.025, -73.675) centre (3.025, -73.175) ccw projected
  line L111 (2.525, -73.175) -> (2.525, -60.175) projected
  arc A75 (3.025, -59.675) -> (2.525, -60.175) centre (3.025, -60.175) ccw projected
  line L112 (41.125, -40.625) -> (54.125, -40.625) projected
  arc A76 (54.625, -41.125) -> (54.125, -40.625) centre (54.125, -41.125) ccw projected
  line L113 (54.625, -41.125) -> (54.625, -54.125) projected
  arc A77 (54.125, -54.625) -> (54.625, -54.125) centre (54.125, -54.125) ccw projected
  line L114 (54.125, -54.625) -> (41.125, -54.625) projected
  arc A78 (40.625, -54.125) -> (41.125, -54.625) centre (41.125, -54.125) ccw projected
  line L115 (40.625, -54.125) -> (40.625, -41.125) projected
  arc A79 (41.125, -40.625) -> (40.625, -41.125) centre (41.125, -41.125) ccw projected
  line L116 (22.075, -40.625) -> (35.075, -40.625) projected
  arc A80 (35.575, -41.125) -> (35.075, -40.625) centre (35.075, -41.125) ccw projected
  line L117 (35.575, -41.125) -> (35.575, -54.125) projected
  arc A81 (35.075, -54.625) -> (35.575, -54.125) centre (35.075, -54.125) ccw projected
  line L118 (35.075, -54.625) -> (22.075, -54.625) projected
  arc A82 (21.575, -54.125) -> (22.075, -54.625) centre (22.075, -54.125) ccw projected
  line L119 (21.575, -54.125) -> (21.575, -41.125) projected
  arc A83 (22.075, -40.625) -> (21.575, -41.125) centre (22.075, -41.125) ccw projected
  line L120 (3.025, -40.625) -> (16.025, -40.625) projected
  arc A84 (16.525, -41.125) -> (16.025, -40.625) centre (16.025, -41.125) ccw projected
  line L121 (16.525, -41.125) -> (16.525, -54.125) projected
  arc A85 (16.025, -54.625) -> (16.525, -54.125) centre (16.025, -54.125) ccw projected
  line L122 (16.025, -54.625) -> (3.025, -54.625) projected
  arc A86 (2.525, -54.125) -> (3.025, -54.625) centre (3.025, -54.125) ccw projected
  line L123 (2.525, -54.125) -> (2.525, -41.125) projected
  arc A87 (3.025, -40.625) -> (2.525, -41.125) centre (3.025, -41.125) ccw projected
  line L124 (60.175, -21.575) -> (73.175, -21.575) projected
  arc A88 (73.675, -22.075) -> (73.175, -21.575) centre (73.175, -22.075) ccw projected
  line L125 (73.675, -22.075) -> (73.675, -35.075) projected
  arc A89 (73.175, -35.575) -> (73.675, -35.075) centre (73.175, -35.075) ccw projected
  line L126 (73.175, -35.575) -> (60.175, -35.575) projected
  arc A90 (59.675, -35.075) -> (60.175, -35.575) centre (60.175, -35.075) ccw projected
  line L127 (59.675, -35.075) -> (59.675, -22.075) projected
  arc A91 (60.175, -21.575) -> (59.675, -22.075) centre (60.175, -22.075) ccw projected
  line L128 (41.125, -21.575) -> (54.125, -21.575) projected
  arc A92 (54.625, -22.075) -> (54.125, -21.575) centre (54.125, -22.075) ccw projected
  line L129 (54.625, -22.075) -> (54.625, -35.075) projected
  arc A93 (54.125, -35.575) -> (54.625, -35.075) centre (54.125, -35.075) ccw projected
  line L130 (54.125, -35.575) -> (41.125, -35.575) projected
  arc A94 (40.625, -35.075) -> (41.125, -35.575) centre (41.125, -35.075) ccw projected
  line L131 (40.625, -35.075) -> (40.625, -22.075) projected
  arc A95 (41.125, -21.575) -> (40.625, -22.075) centre (41.125, -22.075) ccw projected
  line L132 (22.075, -21.575) -> (35.075, -21.575) projected
  arc A96 (35.575, -22.075) -> (35.075, -21.575) centre (35.075, -22.075) ccw projected
  line L133 (35.575, -22.075) -> (35.575, -35.075) projected
  arc A97 (35.075, -35.575) -> (35.575, -35.075) centre (35.075, -35.075) ccw projected
  line L134 (35.075, -35.575) -> (22.075, -35.575) projected
  arc A98 (21.575, -35.075) -> (22.075, -35.575) centre (22.075, -35.075) ccw projected
  line L135 (21.575, -35.075) -> (21.575, -22.075) projected
  arc A99 (22.075, -21.575) -> (21.575, -22.075) centre (22.075, -22.075) ccw projected
  line L136 (3.025, -21.575) -> (16.025, -21.575) projected
  arc A100 (16.525, -22.075) -> (16.025, -21.575) centre (16.025, -22.075) ccw projected
  line L137 (16.525, -22.075) -> (16.525, -35.075) projected
  arc A101 (16.025, -35.575) -> (16.525, -35.075) centre (16.025, -35.075) ccw projected
  line L138 (16.025, -35.575) -> (3.025, -35.575) projected
  arc A102 (2.525, -35.075) -> (3.025, -35.575) centre (3.025, -35.075) ccw projected
  line L139 (2.525, -35.075) -> (2.525, -22.075) projected
  arc A103 (3.025, -21.575) -> (2.525, -22.075) centre (3.025, -22.075) ccw projected
  line L140 (78.581, -121.483) -> (78.581, 13.517) projected
  line L141 (-2.381, 13.517) -> (78.581, 13.517) projected
  line L142 (-2.381, 13.517) -> (-2.381, -121.483) projected
  line L143 (78.581, -121.483) -> (-2.381, -121.483) projected
  line L144 (26.05, -99.8982) -> (27.6606, -99.8982) projected
  line L145 (27.6606, -99.8982) -> (27.6606, -99.5854) projected
  arc A104 (28.1606, -99.0854) -> (27.6606, -99.5854) centre (28.1606, -99.5854) ccw projected
  line L146 (28.1606, -99.0854) -> (33.8154, -99.0854) projected
  arc A105 (34.3154, -99.5854) -> (33.8154, -99.0854) centre (33.8154, -99.5854) ccw projected
  line L147 (34.3154, -99.5854) -> (34.3154, -102.489) projected
  line L148 (34.3154, -102.489) -> (34.679, -102.489) projected
  arc A106 (35.179, -102.989) -> (34.679, -102.489) centre (34.679, -102.989) ccw projected
  line L149 (35.179, -102.989) -> (35.179, -105.283) projected
  line L150 (35.179, -105.283) -> (34.8154, -105.283) projected
  arc A107 (34.8154, -105.283) -> (34.3154, -105.783) centre (34.8154, -105.783) ccw projected
  line L151 (34.3154, -105.783) -> (34.3154, -110.879) projected
  arc A108 (33.8154, -111.379) -> (34.3154, -110.879) centre (33.8154, -110.879) ccw projected
  line L152 (33.8154, -111.379) -> (33.012, -111.379) projected
  arc A109 (33.012, -111.379) -> (32.512, -111.879) centre (33.012, -111.879) ccw projected
  line L153 (32.512, -111.879) -> (32.512, -112.0474) projected
  arc A110 (32.012, -112.5474) -> (32.512, -112.0474) centre (32.012, -112.0474) ccw projected
  line L154 (32.012, -112.5474) -> (29.964, -112.5474) projected
  arc A111 (29.464, -112.0474) -> (29.964, -112.5474) centre (29.964, -112.0474) ccw projected
  line L155 (29.464, -112.0474) -> (29.464, -111.879) projected
  arc A112 (29.464, -111.879) -> (28.964, -111.379) centre (28.964, -111.879) ccw projected
  line L156 (28.964, -111.379) -> (27.6606, -111.379) projected
  line L157 (27.6606, -111.379) -> (27.6606, -111.0916) projected
  arc A113 (27.6606, -111.0916) -> (27.1606, -110.5916) centre (27.1606, -111.0916) ccw projected
  line L158 (27.1606, -110.5916) -> (26.05, -110.5916) projected
  line L159 (26.05, -110.5916) -> (26.05, -111.275) projected
  arc A114 (25.55, -111.775) -> (26.05, -111.275) centre (25.55, -111.275) ccw projected
  line L160 (25.55, -111.775) -> (12.55, -111.775) projected
  arc A115 (12.05, -111.275) -> (12.55, -111.775) centre (12.55, -111.275) ccw projected
  line L161 (12.05, -111.275) -> (12.05, -110.5916) projected
  line L162 (12.05, -110.5916) -> (10.9394, -110.5916) projected
  arc A116 (10.9394, -110.5916) -> (10.4394, -111.0916) centre (10.9394, -111.0916) ccw projected
  line L163 (10.4394, -111.0916) -> (10.4394, -111.379) projected
  line L164 (10.4394, -111.379) -> (9.136, -111.379) projected
  arc A117 (9.136, -111.379) -> (8.636, -111.879) centre (9.136, -111.879) ccw projected
  line L165 (8.636, -111.879) -> (8.636, -112.0474) projected
  arc A118 (8.136, -112.5474) -> (8.636, -112.0474) centre (8.136, -112.0474) ccw projected
  line L166 (8.136, -112.5474) -> (6.088, -112.5474) projected
  arc A119 (5.588, -112.0474) -> (6.088, -112.5474) centre (6.088, -112.0474) ccw projected
  line L167 (5.588, -112.0474) -> (5.588, -111.879) projected
  arc A120 (5.588, -111.879) -> (5.088, -111.379) centre (5.088, -111.879) ccw projected
  line L168 (5.088, -111.379) -> (4.2846, -111.379) projected
  arc A121 (3.7846, -110.879) -> (4.2846, -111.379) centre (4.2846, -110.879) ccw projected
  line L169 (3.7846, -110.879) -> (3.7846, -105.783) projected
  arc A122 (3.7846, -105.783) -> (3.2846, -105.283) centre (3.2846, -105.783) ccw projected
  line L170 (3.2846, -105.283) -> (2.921, -105.283) projected
  line L171 (2.921, -105.283) -> (2.921, -102.989) projected
  arc A123 (3.421, -102.489) -> (2.921, -102.989) centre (3.421, -102.989) ccw projected
  line L172 (3.421, -102.489) -> (3.7846, -102.489) projected
  line L173 (3.7846, -102.489) -> (3.7846, -99.5854) projected
  arc A124 (4.2846, -99.0854) -> (3.7846, -99.5854) centre (4.2846, -99.5854) ccw projected
  line L174 (4.2846, -99.0854) -> (9.9394, -99.0854) projected
  arc A125 (10.4394, -99.5854) -> (9.9394, -99.0854) centre (9.9394, -99.5854) ccw projected
  line L175 (10.4394, -99.5854) -> (10.4394, -99.8982) projected
  line L176 (10.4394, -99.8982) -> (12.05, -99.8982) projected
  line L177 (12.05, -99.8982) -> (12.05, -98.275) projected
  arc A126 (12.55, -97.775) -> (12.05, -98.275) centre (12.55, -98.275) ccw projected
  line L178 (12.55, -97.775) -> (25.55, -97.775) projected
  arc A127 (26.05, -98.275) -> (25.55, -97.775) centre (25.55, -98.275) ccw projected
  line L179 (26.05, -98.275) -> (26.05, -99.8982) projected
  line L180 (60.175, 2.2034) -> (73.175, 2.2034)
  arc A128 (73.675, 1.7034) -> (73.175, 2.2034) centre (73.175, 1.7034) ccw
  line L181 (73.675, 1.7034) -> (73.675, -11.2966)
  arc A129 (73.1684, -11.825) -> (73.675, -11.2966) centre (73.1758, -11.3251) ccw
  line L182 (73.1684, -11.825) -> (60.1684, -11.825)
  arc A130 (59.675, -11.2966) -> (60.1684, -11.825) centre (60.1742, -11.325) ccw
  line L183 (59.675, -11.2966) -> (59.675, 1.7034)
  arc A131 (60.175, 2.2034) -> (59.675, 1.7034) centre (60.175, 1.7034) ccw
  point P0 (0, 0)
  dimension "d34" = 0
  dimension "d35" = 0
  dimension "d36" = 13
  dimension "d39" = 9.75
  constraints: 8 end point, 8 point on circle, 4 centre point
  measures "d34" distance between parallel lines of L183 L127
  measures "d35" distance between parallel lines of L125 L181
  measures "d36" distance of L180.start L180.end
  measures "d39" distance between parallel lines of L124 L182
extrude "Extrusion7" cut sketch "Sketch12" against normal blind 7.183 contours L180 A128 L181 A129 L182 A130 L183 A131
sketch "Sketch14" plane through (0, 0, 1.6) normal (0, 0, 1) x (1, 0, 0)
  line L0 (67.425, 6.6474) -> (71.625, 6.6474)
  line L1 (71.625, 6.6474) -> (71.625, 4.4474)
  line L2 (71.625, 4.4474) -> (67.425, 4.4474)
  line L3 (67.425, 4.4474) -> (67.425, 6.6474)
  line L4 (43.625, -5.662) -> (45.825, -5.662)
  line L5 (45.825, -5.662) -> (45.825, -9.862)
  line L6 (45.825, -9.862) -> (43.625, -9.862)
  line L7 (43.625, -9.862) -> (43.625, -5.662)
  line L8 (42.314, -0.408) -> (42.314, -9.117) projected
  line L9 (42.314, -9.117) -> (29.113, -9.117) projected
  arc A0 (73.675, 1.7034) -> (73.175, 2.2034) centre (73.175, 1.7034) ccw projected
  point P0 (0, 0)
  dimension "d40" = 1.311
  dimension "d41" = 2.2
  dimension "d42" = 4.2
  dimension "d43" = 0.745
  dimension "d44" = 1.55
  dimension "d45" = 2.244
  dimension "d46" = 4.2
  dimension "d47" = 2.2
  constraints: 16 end point, 4 parallel, 2 horizontal, 2 perpendicular
  measures "d40" distance between parallel lines of L8 L7
  measures "d41" distance between parallel lines of L5 L7
  measures "d42" distance between parallel lines of L6 L4
  measures "d43" distance between parallel lines of L6 L9
  measures "d44" distance from line of L1 A0.end
  measures "d45" distance from line of A0.end L2
  measures "d46" distance between parallel lines of L3 L1
  measures "d47" distance between parallel lines of L2 L0
extrude "Extrusion8" cut sketch "Sketch14" against normal blind 10
fillet "Fillet1" radius 2 4 edges at (78.581, 13.517, 0.8) (-2.381, 13.517, 0.8) (78.581, -121.483, 0.8) (-2.381, -121.483, 0.8)
sketch "Sketch15" plane through (0, 0, 0) normal (0, 0, -1) x (-1, 0, 0)
  line L0 (0.381, 13.517) -> (-76.581, 13.517) projected
  line L1 (-63.887, 17.707) -> (-63.887, 13.517)
  line L2 (-63.887, 17.707) -> (-47.087, 17.707)
  line L3 (-47.087, 17.707) -> (-47.087, 13.517)
  line L4 (-63.887, 13.517) -> (-47.087, 13.517)
  line L5 (0.381, -121.483) -> (-76.581, -121.483) projected
  line L6 (-63.887, -121.483) -> (-63.887, -124.633)
  line L7 (-63.887, -124.633) -> (-12.362, -124.633)
  line L8 (-12.362, -124.633) -> (-12.362, -121.483)
  line L9 (-63.887, -121.483) -> (-12.362, -121.483)
  point P0 (0, 0)
  dimension "d51" = 12.694
  dimension "d52" = 4.19
  dimension "d53" = 16.8
  dimension "d54" = 3.15
  dimension "d55" = 12.694
  dimension "d56" = 51.525
  constraints: 16 end point, 4 point on line, 3 perpendicular, 2 collinear, 2 horizontal, 1 coincident, 1 vertical
  measures "d51" horizontal distance of L1.start L0.end
  measures "d52" distance from line of L0 L1.start
  measures "d53" distance of L1.start L2.end
  measures "d54" distance of L6.start L6.end
  measures "d55" distance from line of L6 point (-76.581, -121.483)
  measures "d56" distance of L6.end L7.end
extrude "Extrusion9" add sketch "Sketch15" against normal up to surface (1.6 mm away)
body "Solid1"
